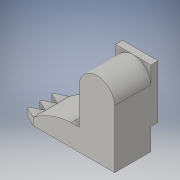
# Autodesk Inventor part: Leg
Saved by Autodesk Inventor 2016 (Build 200138000, 138)
## iProperties
Created: 2017-03-12
Part Number: Leg
Material: Generic
Document SubType Name: Modeling
Designer: Owner
Density: 1 g/cm^3
Appearance: Default
Author: Owner
Autodesk Inventor part; units mm, degrees
ref_plane "YZ Plane" through (0, 0, 0) normal (1, 0, 0) x (0, 1, 0)
ref_plane "XZ Plane" through (0, 0, 0) normal (0, 1, 0) x (-1, 0, 0)
ref_plane "XY Plane" through (0, 0, 0) normal (0, 0, 1) x (1, 0, 0)
sketch "Sketch1" plane through (0, 0, 0) normal (0, 0, 1) x (1, 0, 0)
  line L0 (46.95, 0) -> (46.95, 38.1) projected
  line L1 (46.95, 38.1) -> (59.65, 38.1) projected
  line L2 (59.65, 38.1) -> (72.35, 38.1) projected
  line L3 (72.35, 38.1) -> (72.35, 0) projected
  circle A0 centre (61.35, -6.35) radius 12.065 projected
  line L4 (46.95, 38.1) -> (47.2, 38.1)
  line L5 (47.2, 38.1) -> (47.2, 37.85)
  line L6 (72.35, 0) -> (72.1, 0)
  line L7 (72.1, 0) -> (72.1, 0.25)
  line L8 (72.1, 0.25) -> (47.2, 0.25)
  line L9 (47.2, 0.25) -> (47.2, 37.85)
  line L10 (47.2, 37.85) -> (72.1, 37.85)
  line L11 (72.1, 37.85) -> (72.1, 0.25)
  point P0 (0, 0)
  dimension "d0" = 0.25
  dimension "d1" = 0.25
  dimension "d2" = 0.25
  dimension "d3" = 0.25
  constraints: 16 end point, 3 perpendicular, 2 horizontal, 2 parallel, 1 point on line
  measures "d0" distance of L0.end L4.end
  measures "d1" distance of L4.end L5.end
  measures "d2" distance of L3.end L6.end
  measures "d3" distance of L6.end L7.end
extrude "Extrusion1" add sketch "Sketch1" against normal blind 5 contours L10 L11 L8 A0 L9 | A0 L8 picked at (62.9802, 2.7077)
sketch "Sketch2" plane through (0, 0, 0) normal (0, 0, 1) x (1, 0, 0)
  line L0 (47.2, 37.85) -> (72.1, 37.85) projected
  line L1 (47.2, 37.85) -> (47.2, 12.958)
  line L2 (72.1, 37.85) -> (72.1, 0.25) projected
  circle A0 centre (59.6397, 25.404) radius 12.446
  line L3 (47.2, 0.25) -> (47.2, 37.85) projected
  line L4 (47.2, 25.7997) -> (72.1, 25.7997)
  line L5 (72.1, 25.7997) -> (72.1, 0.25)
  line L6 (72.1, 0.25) -> (47.2, 0.25)
  line L7 (47.2, 0.25) -> (47.2, 25.7997)
  point P0 (0, 0)
  dimension "d6" = 24.892
  constraints: 10 end point, 3 parallel, 2 horizontal, 1 perpendicular, 1 point on line, 3 other
  measures "d6" distance of L0.start L1.end
extrude "Extrusion2" add sketch "Sketch2" along normal blind 25.4 contours A0 L4 | L4 A0 L1 | L1 A0 | L4 L2 L6 L3 L1 A0
sketch "Sketch3" plane through (0, 0, 25.4) normal (0, 0, 1) x (1, 0, 0)
  circle A0 centre (61.35, -6.35) radius 12.065 projected
  circle A1 centre (61.35, -6.35) radius 6.35 projected
  line L0 (72.1, 37.85) -> (72.1, 0.25) projected
  line L1 (72.1, 0.25) -> (14.95, 0.25)
  line L2 (14.95, 0.25) -> (14.95, -14.99)
  line L3 (14.95, -14.99) -> (72.1, -14.99)
  line L4 (72.1, -14.99) -> (72.1, 0.25)
  line L5 (14.95, 0.25) -> (72.1, 0.25)
  line L6 (72.1, 0.25) -> (72.1, 10.41)
  point P0 (0, 0)
  dimension "d9" = 15.24
  dimension "d10" = 57.15
  constraints: 12 end point, 2 horizontal, 2 parallel, 2 perpendicular, 1 point on line
  measures "d9" distance of L1.end L2.end
  measures "d10" distance of L2.end L3.end
extrude "Extrusion3" add sketch "Sketch3" against normal blind 25.4 contours L4 A0 L3 L1 | A0 L1 L4 | L4 L3 A0 | A0 L3 L2 L1 | A1
sketch "Sketch5" plane through (72.1, -14.99, 0) normal (0, -1, 0) x (1, 0, 0)
  line L0 (-57.15, 25.4) -> (-57.15, 0) projected
  line L1 (-65.6167, 4.2333) -> (-57.15, 0)
  line L2 (-65.6167, 4.2333) -> (-57.15, 8.4667)
  line L3 (-65.6167, 21.1667) -> (-57.15, 25.4)
  line L4 (-65.6167, 21.1667) -> (-57.15, 16.9333)
  line L5 (-57.15, 16.9333) -> (-65.6167, 12.7)
  line L6 (-65.6167, 12.7) -> (-57.15, 8.4667)
  line L7 (0, 25.4) -> (0, 0) projected
  line L8 (-57.15, 25.4) -> (0, 25.4)
  line L9 (0, 25.4) -> (0, 0)
  line L10 (0, 0) -> (-57.15, 0)
  line L11 (0, 0) -> (-57.15, 0) projected
  line L12 (-57.15, 0) -> (-65.6167, 4.2333)
  line L13 (-65.6167, 4.2333) -> (-57.15, 8.4667)
  line L14 (-57.15, 8.4667) -> (-65.6167, 12.7)
  line L15 (-65.6167, 12.7) -> (-57.15, 16.9333)
  line L16 (-57.15, 16.9333) -> (-65.6167, 21.1667)
  line L17 (-65.6167, 21.1667) -> (-57.15, 25.4)
  point P0 (-72.1, 0)
  dimension "d16" = 8.4667
  constraints: 30 end point, 4 equal length, 2 point on line, 1 horizontal, 1 perpendicular
  measures "d16" distance of L0.end L2.end
extrude "Extrusion5" add sketch "Sketch5" against normal blind 5.08
sketch "Sketch6" plane through (0, 0, 25.4) normal (0, 0, 1) x (1, 0, 0)
  line L0 (14.95, 0.25) -> (14.95, -9.91) projected
  line L1 (14.95, -9.91) -> (14.95, 0.25)
  line L2 (14.95, 0.25) -> (47.2, 0.25)
  arc A0 (47.2, 0.25) -> (14.95, -9.91) centre (44.4515, -47.2897) ccw
  point P0 (0, 0)
  point P1 (41.7029, 0.25)
  constraints: 4 end point, 3 point on circle, 1 centre point, 1 perpendicular, 1 point on line, 1 vertical
extrude "Extrusion6" cut sketch "Sketch6" against normal blind 2540 contours L2 A0 L0
ref_plane "Work Plane1" through (0, 0, 12.7) normal (0, 0, 1) x (1, 0, 0)
sketch "Sketch7" plane through (0, 0, 12.7) normal (0, 0, 1) x (1, 0, 0)
  circle A0 centre (61.4402, -11.9143) radius 6.5 projected
  line L0 (61.4402, -5.4143) -> (61.4402, -4.4143)
  line L1 (61.4402, -4.4143) -> (54.9402, -4.4143)
  line L2 (54.9402, -4.4143) -> (53.9402, -4.4143)
  line L3 (53.9402, -4.4143) -> (53.9402, -14.99)
  line L4 (14.95, -14.99) -> (72.1, -14.99) projected
  line L5 (53.9402, -14.99) -> (67.9402, -14.99)
  line L6 (67.9402, -14.99) -> (68.9402, -14.99)
  line L7 (68.9402, -14.99) -> (68.9402, -4.4143)
  line L8 (68.9402, -4.4143) -> (53.9402, -4.4143)
  line L9 (53.9402, -4.4143) -> (68.9402, -4.4143)
  line L10 (68.9402, -4.4143) -> (68.9402, -14.99)
  line L11 (68.9402, -14.99) -> (53.9402, -14.99)
  line L12 (53.9402, -14.99) -> (53.9402, -4.4143)
  point P0 (0, 0)
  dimension "d27" = 1
  dimension "d28" = 1
  dimension "d29" = 1
  constraints: 24 end point, 5 perpendicular, 5 point on line, 2 parallel, 1 horizontal, 1 vertical, 1 vertical alignment, 1 other
  measures "d27" distance of L0.start L0.end
  measures "d28" distance of L1.end L2.end
  measures "d29" distance of L5.end L6.end
extrude "Extrusion7" cut sketch "Sketch7" along normal mid plane 6 contours A0 L4 | A0 L0 L8 L7 L4 | A0 L4 L3 L2 L1 L0 picked at (61.4402, -11.7981)
sketch "Sketch8" plane through (0, 0, 0) normal (0, 0, -1) x (-1, 0, 0)
  circle A0 centre (-61.4402, -11.9143) radius 2 projected
  circle A1 centre (-61.4402, -11.9143) radius 1.75
  point P0 (0, 0)
  dimension "d34" = 3.5
  constraints: 1 centre point, 1 coincident
  measures "d34" diameter of A1
extrude "Extrusion8" cut sketch "Sketch8" against normal blind 12.7 contours A1
sketch "Sketch9" plane through (0, 0, 0) normal (0, 0, -1) x (-1, 0, 0)
  line L0 (-53.9402, -14.99) -> (-68.9402, -14.99) projected
  line L1 (-61.4402, -14.99) -> (-66.4402, -14.99)
  line L2 (-61.4402, -14.99) -> (-56.4402, -14.99)
  line L3 (-56.4402, -14.99) -> (-56.4402, -10.1643)
  circle A0 centre (-61.4402, -11.9143) radius 1.75 projected
  line L4 (-56.4402, -11.9143) -> (-56.4402, -8.8385)
  line L5 (-56.4402, -8.8385) -> (-66.4402, -8.8385)
  line L6 (-66.4402, -8.8385) -> (-66.4402, -14.99)
  point P0 (0, 0)
  dimension "d35" = 5
  dimension "d36" = 5
  dimension "d37" = 3.0757
  dimension "d38" = 3.0757
  constraints: 12 end point, 3 perpendicular, 2 point on line, 1 collinear, 1 midpoint, 1 vertical
  measures "d35" distance of L1.start L1.end
  measures "d36" distance of L1.start L2.end
  measures "d37" distance from line of L0 A0.centre
  measures "d38" distance of L4.start L4.end
extrude "Extrusion9" cut sketch "Sketch9" against normal blind 5
sketch "Sketch10" plane through (0, 0, 15.7) normal (0, 0, -1) x (-1, 0, 0)
  circle A0 centre (-61.4402, -11.9143) radius 2 projected
  circle A1 centre (-61.4402, -11.9143) radius 1.75 projected
  point P0 (0, 0)
extrude "Extrusion10" cut sketch "Sketch10" against normal blind 5 contours A1
fillet "Fillet1" radius 0.5 3 edges at (6.4833, -12.45, 4.2333) (6.4833, -12.45, 12.7) (6.4833, -12.45, 21.1667)
equation "\"d38\" = d37"
body "Solid1"
